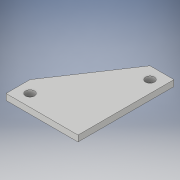
# Autodesk Inventor part: 15102898-16-P-0213
Saved by Autodesk Inventor 2017 (Build 210142000, 142)
## iProperties
Created: 2016-10-05
Part Number: 15102898-16-P-0213
Material: Generic
Document SubType Name: Modeling
Designer: gus
Density: 1 g/cm^3
Appearance: Default
Author: gus
Autodesk Inventor part; units mm, degrees
ref_plane "YZ Plane" through (0, 0, 0) normal (1, 0, 0) x (0, 1, 0)
ref_plane "XZ Plane" through (0, 0, 0) normal (0, 1, 0) x (-1, 0, 0)
ref_plane "XY Plane" through (0, 0, 0) normal (0, 0, 1) x (1, 0, 0)
sketch "Sketch1" plane through (0, 0, 0) normal (0, 1, 0) x (-1, 0, 0)
  line L0 (0, 0) -> (25.4, 0)
  line L1 (25.4, -101.6) -> (0, -101.6)
  line L2 (0, -101.6) -> (0, 0)
  circle A0 centre (63.5, -12.7) radius 4.7625
  circle A1 centre (12.7, -88.9) radius 4.7625
  line L3 (25.4, -101.6) -> (76.2, -25.4)
  line L4 (76.2, -25.4) -> (76.2, 0)
  line L5 (76.2, 0) -> (0, 0)
  dimension "d0" = 25.4
  dimension "d1" = 101.6
  dimension "d2" = 9.525
  dimension "d3" = 9.525
  dimension "d4" = 12.7
  dimension "d6" = 12.7
  dimension "d7" = 12.7
  dimension "d10" = 25.4
  dimension "d11" = 76.2
  dimension "d12" = 12.7
  constraints: 12 end point, 2 centre point, 1 collinear, 1 horizontal, 1 parallel, 1 vertical
  measures "d0" distance of L1.start L1.end
  measures "d1" distance of L0.end L1.start
  measures "d2" diameter of A0
  measures "d3" diameter of A1
  measures "d4" distance from line of L2 A1.centre
  measures "d6" distance from line of L1 A1.centre
  measures "d7" distance from line of L0 A0.centre
  measures "d10" distance of L3.end L4.end
  measures "d11" distance of L4.end L0.start
  measures "d12" distance from line of L4 A0.centre
extrude "Extrusion1" add sketch "Sketch1" along normal blind 6.35
body "Solid1"
